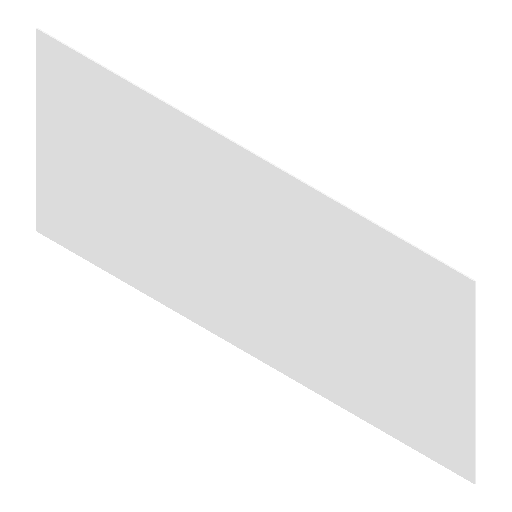
# Autodesk Inventor part: BUY - Cover glass - 24 x 60 x 0.17
Saved by Autodesk Inventor 2025.3 (Build 293356000, 356)
## iProperties
Part Number: BUY - Cover glass - 24 x 60 x 0.17
Material: Generic
Description: Cover glass 24 x 60 mm, 0.17 mm
Document SubType Name: Modeling
Designer: benir
Appearance: Clear - Light
Author: benir
Autodesk Inventor part; units mm, degrees
ref_plane "YZ Plane" through (0, 0, 0) normal (1, 0, 0) x (0, 1, 0)
ref_plane "XZ Plane" through (0, 0, 0) normal (0, 1, 0) x (-1, 0, 0)
ref_plane "XY Plane" through (0, 0, 0) normal (0, 0, 1) x (1, 0, 0)
sketch "glass sketch" plane through (0, 0, 0) normal (0, 0, 1) x (1, 0, 0)
  line L0 (-30, -12) -> (30, -12)
  line L1 (30, -12) -> (30, 12)
  line L2 (30, 12) -> (-30, 12)
  line L3 (-30, 12) -> (-30, -12)
  line L4 (0, -16.8) -> (0, 16.8) projected
  line L5 (-42, 0) -> (42, 0) projected
  dimension "d0" = 60
  dimension "d1" = 24
  constraints: 8 end point, 2 parallel, 1 horizontal, 1 perpendicular, 2 other
  measures "d0" distance of L0.start L0.end
  measures "d1" distance of L2.end L0.start
extrude "glass" add sketch "glass sketch" against normal blind 0.17
equation "\"d0\" = glass_l"
equation "\"d1\" = glass_w"
equation "\"d2\" = glass_t"
equation "\"glass_l\" = 60"
equation "\"glass_w\" = 24"
equation "\"glass_t\" = 0.17"
body "Solid1"
